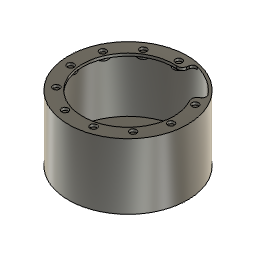
BatteryPack v8 (Autodesk Fusion 360 design; units mm, degrees)
Autodesk Fusion 360 part; units mm, degrees
sketch "Sketch1" plane through (0, 0, 0) normal (0, 0, 1) x (1, 0, 0)
  circle A0 centre (0, 0) radius 44.5
  circle A1 centre (0, 0) radius 42.5
  dimension "d1" = 89
  dimension "d2" = 2
  constraint coincident A0.centre A1.centre
  measures "d1" diameter of A0
  measures "d2" distance of A0 A1
extrude "Extrude1" add sketch "Sketch1" against normal blind 2 contours A0 | A1 makes body 1
extrude "Extrude2" add sketch "Sketch1" along normal blind 45 bodies 1
sketch "Sketch2" plane through (0, 0, 45) normal (0, 0, 1) x (-1, 0, 0)
  circle A0 centre (0, 0) radius 42.5
  circle A1 centre (0, 0) radius 44.5
  circle A2 centre (0, 0) radius 44.5
  dimension "d7" = 89
  constraint concentric A0 A2
  measures "d7" diameter of A2
extrude "Extrude3" add sketch "Sketch2" along normal blind 2 separate body contours A0 | A1 A2 makes body 2
sketch "Sketch3" plane through (0, 0, 47) normal (0, 0, 1) x (-1, 0, 0)
  circle A0 centre (0, 0) radius 44.5
  circle A1 centre (0, -38) radius 2.5
  circle A2 centre (0, -38) radius 4
  dimension "d10" = 5
  dimension "d12" = 1.5
  dimension "d24" = 38
  constraint concentric A1 A2
  constraint vertical A0.centre A1.centre
  measures "d10" diameter of A1
  measures "d12" distance of A1 A2
  measures "d24" distance of A0.centre A1.centre
extrude "Extrude4" add sketch "Sketch3" against normal blind 3.5 contours A1 | A2 bodies 2
extrude "Extrude5" cut sketch "Sketch3" against normal blind 2 contours A1 bodies 2
pattern_circular "C-Pattern1" count 11 over 360 about axis through (0, 0, 1.75) along (0, 0, 1) of "Extrude4", "Extrude5"
sketch "Sketch5" plane through (0, 0, 47) normal (0, 0, 1) x (-1, 0, 0)
  circle A0 centre (10.7058, 36.4607) radius 2.5
  circle A1 centre (28.7185, 24.8847) radius 2.5
  circle A2 centre (37.6132, 5.408) radius 2.5
  circle A3 centre (34.566, -15.7858) radius 2.5
  circle A4 centre (20.5444, -31.9676) radius 2.5
  circle A5 centre (0, -38) radius 2.5
  circle A6 centre (0, 0) radius 44.5
  circle A7 centre (0, 0) radius 34
  circle A8 centre (0, -38) radius 4
  circle A9 centre (-37.6132, 5.408) radius 2.5
  circle A10 centre (-28.7185, 24.8847) radius 2.5
  circle A11 centre (-10.7058, 36.4607) radius 2.5
  circle A12 centre (-34.566, -15.7858) radius 2.5
  circle A13 centre (-20.5444, -31.9676) radius 2.5
  constraint concentric A6 A7
  constraint tangent A7 A8
extrude "Extrude6" cut sketch "Sketch5" against normal blind 5 contours A7 bodies 2
sketch "Sketch7" plane through (0, 0, 47) normal (0, 0, 1) x (-1, 0, 0)
  circle A0 centre (0, 0) radius 34
  circle A1 centre (10.7058, 36.4607) radius 2.5
  circle A2 centre (28.7185, 24.8847) radius 2.5
  circle A3 centre (37.6132, 5.408) radius 2.5
  circle A4 centre (34.566, -15.7858) radius 2.5
  circle A5 centre (20.5444, -31.9676) radius 2.5
  circle A6 centre (0, -38) radius 2.5
  circle A7 centre (0, 0) radius 44.5
  arc A8 (41.3317, -9.8965) -> (42.4456, -2.1489) centre (0, 0) ccw
  arc A9 (34.5241, -8.2665) -> (41.3317, -9.8965) centre (37.9279, -9.0815) ccw
  arc A10 (34.5241, -8.2665) -> (35.4546, -1.795) centre (0, 0) ccw
  arc A11 (42.4456, -2.1489) -> (35.4546, -1.795) centre (38.9501, -1.9719) ccw
  arc A12 (37.9279, -9.0815) -> (38.9501, -1.9719) centre (0, 0) ccw construction
  circle A13 centre (-37.6132, 5.408) radius 2.5
  circle A14 centre (-28.7185, 24.8847) radius 2.5
  circle A15 centre (-10.7058, 36.4607) radius 2.5
  circle A16 centre (-34.566, -15.7858) radius 2.5
  circle A17 centre (34.566, -15.7858) radius 4
  circle A18 centre (37.6132, 5.408) radius 4
  circle A19 centre (-20.5444, -31.9676) radius 2.5
  dimension "d25" = 2
  dimension "d26" = 39
  constraint tangent A8 A9
  constraint tangent A9 A10
  constraint tangent A10 A11
  constraint tangent A8 A11
  constraint coincident A0.centre A7.centre
  constraint tangent A9 A17
  constraint tangent A11 A18
  measures "d25" distance of A7 A8
  measures "d26" radius of A12
combine "Combine1" operation add target body 1 tool bodies 2
sketch "Sketch9" plane through (0, 0, 47) normal (0, 0, 1) x (-1, 0, 0)
  circle A0 centre (0, 0) radius 44.5 construction
  line L0 (0, 0) -> (-7.973, -43.7799)
  line L1 (0, 0) -> (-36.5115, -25.4393)
  circle A1 centre (0, 0) radius 34 construction
  circle A2 centre (0, 0) radius 42.5
  circle A3 centre (28.7185, 24.8847) radius 4
  circle A4 centre (10.7058, 36.4607) radius 4
  constraint coincident A0.centre L0.start
  constraint coincident A0 L0.end
  constraint coincident A0 L1.end
  constraint tangent L1 A3
  constraint tangent L0 A4
extrude "Extrude8" cut sketch "Sketch9" against normal blind 6 contours L0 L1 A2 picked at (-13.7041, -24.73) bodies 1
fillet "Fillet1" radius 4 2 edges at (6.0917, 33.4498, 46) (27.8964, 19.4368, 46) on bodies 1
fillet "Fillet2" radius 3 2 edges at (7.6146, 41.8123, 46) (34.8706, 24.296, 46) on bodies 1
